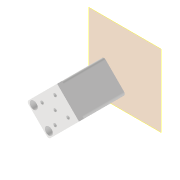
# Autodesk Inventor part: IM_ledmatrix_holder
Saved by Autodesk Inventor 2022 (Build 260153000, 153)
## iProperties
Created: 2023-06-20
Part Number: IM_ledmatrix_holder
Material: Generisch
Document SubType Name: Modeling
Designer: diederichbenedict
Density: 1 g/cm^3
Appearance: Vorgabe
Author: diederichbenedict
Autodesk Inventor part; units mm, degrees
ref_plane "YZ Plane" through (0, 0, 0) normal (1, 0, 0) x (0, 1, 0)
ref_plane "XZ Plane" through (0, 0, 0) normal (0, 1, 0) x (-1, 0, 0)
ref_plane "XY Plane" through (0, 0, 0) normal (0, 0, 1) x (1, 0, 0)
ref_plane "Arbeitsebene1" through (0, 0, 0) normal (0, 0, 1) x (1, 0, 0)
sketch "Skizze1" plane through (0, 0, 0) normal (0, 0, 1) x (1, 0, 0)
  circle A0 centre (-5.0971, -17.293) radius 1.4
  circle A1 centre (-17.4192, -5.2278) radius 1.4
  arc A2 (5.6957, 26.2674) -> (7.9686, 25.6694) centre (6.0612, 23.038) ccw
  arc A3 (5.6957, 26.2674) -> (-18.8161, -19.193) centre (0, 0) ccw
  arc A4 (-18.1702, -19.8055) -> (-18.8161, -19.193) centre (-16.2778, -17.1634) ccw
  arc A5 (-18.1702, -19.8055) -> (25.9554, 6.9811) centre (0, 0) ccw
  arc A6 (25.2463, 9.2218) -> (25.9554, 6.9811) centre (22.7119, 7.1872) ccw
  arc A7 (25.2463, 9.2218) -> (7.9686, 25.6694) centre (0, 0) ccw
  spline S0 degree 3 poles (-11.5553, -6.2972) (-11.3711, -6.4814) (-11.2247, -6.6998) (-11.0238, -7.1803) (-10.9713, -7.4379) (-10.9679, -7.9586) (-11.0171, -8.2168) (-11.2083, -8.6915) (-11.3454, -8.905) (-11.5184, -9.0874) knots 0 0 0 0 0.252225 0.252225 0.504373 0.504373 0.756494 0.756494 1 1 1 1
  line L0 (-11.5553, -6.2972) -> (-16.3497, -1.5028)
  arc A8 (-16.3497, 1.4985) -> (-16.3497, -1.5028) centre (-14.8491, -0.0022) ccw
  line L1 (-16.3497, 1.4985) -> (-1.5005, 16.3477)
  arc A9 (1.5007, 16.3477) -> (-1.5005, 16.3477) centre (0.0001, 14.8471) ccw
  line L2 (1.5007, 16.3477) -> (16.35, 1.4985)
  arc A10 (16.35, -1.5028) -> (16.35, 1.4985) centre (14.8494, -0.0022) ccw
  line L3 (16.35, -1.5028) -> (1.5007, -16.352)
  arc A11 (-1.5005, -16.352) -> (1.5007, -16.352) centre (0.0001, -14.8514) ccw
  line L4 (-1.5005, -16.352) -> (-4.7949, -13.0576)
  spline S1 degree 3 poles (-7.585, -13.0208) (-7.3961, -12.8415) (-7.1739, -12.7009) (-6.6882, -12.5128) (-6.4293, -12.4671) (-5.9087, -12.4775) (-5.6519, -12.5335) (-5.1824, -12.7372) (-4.9727, -12.8798) (-4.7949, -13.0576) knots 0 0 0 0 0.252231 0.252231 0.504388 0.504388 0.756517 0.756517 1 1 1 1
  arc A12 (-11.5184, -9.0874) -> (-7.585, -13.0208) centre (-9.4998, -11.0022) ccw
  line L5 (-17.4192, -5.2278) -> (-5.0971, -17.293)
  line L6 (-17.8503, -0.0022) -> (0.0001, -17.8526)
  line L7 (0.0001, -17.8526) -> (-3.889, -21.7417)
  line L8 (-6.7174, -21.7417) -> (-21.7394, -6.7197)
  line L9 (-21.7394, -3.8912) -> (-17.8503, -0.0022)
  arc A13 (-21.7394, -3.8912) -> (-21.7394, -6.7197) centre (-20.3252, -5.3055) ccw
  arc A14 (-6.7174, -21.7417) -> (-3.889, -21.7417) centre (-5.3032, -20.3275) ccw
  line L10 (-17.8503, -0.0022) -> (-18.5575, -0.7093)
  line L11 (-15.729, -0.7093) -> (-0.707, -15.7313)
  line L12 (-0.707, -18.5597) -> (0.0001, -17.8526)
  line L13 (0.0001, -17.8526) -> (-17.8503, -0.0022)
  arc A15 (-15.729, -0.7093) -> (-18.5575, -0.7093) centre (-17.1432, -2.1235) ccw
  arc A16 (-0.707, -18.5597) -> (-0.707, -15.7313) centre (-2.1212, -17.1455) ccw
  point P0 (0, 0)
  point P1 (-5.3032, -23.1559)
  point P2 (-11.5553, -6.2972)
  point P3 (-1.5005, -16.352)
  point P4 (-17.1432, 0.705)
  dimension "d0" = 7.5
  dimension "d1" = 2
  dimension "d23" = 1
  dimension "d24" = 2
  constraints: 18 end point, 8 point on circle, 8 tangent, 4 centre point, 4 parallel, 4 point on line, 3 perpendicular, 2 equal radius
  measures "d0" distance of L6.end point (-5.303, -23.156)
  measures "d1" radius of A13
  measures "d23" distance of L6.start point (-17.143, 0.705)
  measures "d24" radius of A15
extrude "Extrusion1" add sketch "Skizze1" along normal blind 50 contours L6 S1 A12 L5 S0 | S0 A12 S1 L4 L6 A16 L7 A14 L8 A13 L9 A15 L0 | L0 A8 A15 L11 A16 A11 L4 L6 | L6 A15 A8 | L5 A12 | A11 A16 L6
sketch "Skizze2" plane through (0, 0, 50) normal (0, 0, 1) x (1, 0, 0)
  line L0 (-21.2132, 0) -> (0, -21.2132) projected
  line L1 (-18.5575, -0.7093) -> (-21.7394, -3.8912) projected
  arc A0 (-21.7394, -3.8912) -> (-21.7394, -6.7197) centre (-20.3252, -5.3055) ccw projected
  line L2 (-21.7394, -6.7197) -> (-6.7174, -21.7417) projected
  arc A1 (-6.7174, -21.7417) -> (-3.889, -21.7417) centre (-5.3032, -20.3275) ccw projected
  line L3 (-3.889, -21.7417) -> (-0.707, -18.5597) projected
  circle A2 centre (-17.4192, -5.2278) radius 1.4 projected
  circle A3 centre (-5.0971, -17.293) radius 1.4 projected
  arc A4 (-0.707, -18.5597) -> (-0.707, -15.7313) centre (-2.1212, -17.1455) ccw projected
  line L4 (-0.707, -15.7313) -> (-15.729, -0.7093) projected
  arc A5 (-15.729, -0.7093) -> (-18.5575, -0.7093) centre (-17.1432, -2.1235) ccw projected
  point P0 (0, 0)
  point P1 (-1.6802, -19.533)
  point P2 (-3.7126, -17.5006)
  point P3 (-5.3048, -15.9084)
  point P4 (-16.0196, -5.1936)
  point P5 (-17.385, -3.8282)
  point P6 (-19.5307, -1.6825)
extrude "Extrusion2" add sketch "Skizze2" along normal blind 4 contours L0 A2 A3 L3 A1 L2 A0 L1
sketch "Skizze3" plane through (0, 0, 54) normal (0, 0, 1) x (1, 0, 0)
  line L0 (21.2132, 0) -> (0, 21.2132) projected
  line L1 (0, 21.2132) -> (-21.2132, 0) projected
  line L2 (-21.2132, 0) -> (0, -21.2132) projected
  line L3 (0, -21.2132) -> (21.2132, 0) projected
  circle A0 centre (0, 0) radius 1.3301 projected
  circle A1 centre (-10.6066, 0) radius 1.5 projected
  circle A2 centre (0, -10.6066) radius 1.5 projected
  circle A3 centre (10.6066, 0) radius 1.5 projected
  circle A4 centre (0, 10.6066) radius 1.5 projected
  line L4 (-3.889, -21.7417) -> (-1.6802, -19.533) projected
  line L5 (-1.6802, -19.533) -> (-3.7126, -17.5006) projected
  arc A5 (-5.3048, -15.9084) -> (-3.7126, -17.5006) centre (-5.0971, -17.293) ccw projected
  line L6 (-5.3048, -15.9084) -> (-16.0196, -5.1936) projected
  arc A6 (-17.385, -3.8282) -> (-16.0196, -5.1936) centre (-17.4192, -5.2278) ccw projected
  line L7 (-17.385, -3.8282) -> (-19.5307, -1.6825) projected
  line L8 (-19.5307, -1.6825) -> (-21.7394, -3.8912) projected
  arc A7 (-21.7394, -3.8912) -> (-21.7394, -6.7197) centre (-20.3252, -5.3055) ccw projected
  line L9 (-21.7394, -6.7197) -> (-6.7174, -21.7417) projected
  arc A8 (-6.7174, -21.7417) -> (-3.889, -21.7417) centre (-5.3032, -20.3275) ccw projected
  arc A9 (-16.0196, -5.1936) -> (-17.385, -3.8282) centre (-17.4192, -5.2278) ccw projected
  arc A10 (-3.7126, -17.5006) -> (-5.3048, -15.9084) centre (-5.0971, -17.293) ccw projected
  circle A11 centre (-10.6066, 0) radius 1.4
  circle A12 centre (0, 10.6066) radius 1.4
  circle A13 centre (10.6066, 0) radius 1.4
  circle A14 centre (0, -10.6066) radius 1.4
  line L10 (-19.5307, -1.6825) -> (1.6825, 19.5307)
  line L11 (-1.6802, -19.533) -> (19.533, 1.6802)
  point P0 (0, 0)
  dimension "d14" = 2.8
  dimension "d15" = 2.8
  dimension "d16" = 2.8
  dimension "d17" = 2.8
  constraints: 4 centre point, 4 coincident, 4 end point, 2 perpendicular, 2 point on line
  measures "d14" diameter of A11
  measures "d15" diameter of A12
  measures "d16" diameter of A13
  measures "d17" diameter of A14
extrude "Extrusion3" add sketch "Skizze3" along normal blind 4 contours L11 L2 A10 A9 L10 L0 | L4 A8 L9 A7 L8 L2 A6 A5 | A1 | A2 | A3 | A4
sketch "Skizze4" plane through (0.0001, -17.8526, 50) normal (0.7071068, -0.7071068, 0) x (-0.7071068, -0.7071068, 0)
  line L0 (5.5, 50) -> (1, 50) projected
  line L1 (2.3764, 0) -> (1, 0) projected
  line L2 (2.3764, 0) -> (2.3764, -4) projected
  line L3 (5.5, -8) -> (-27.6236, -8) projected
  line L4 (5.5, 50) -> (5.5, -8) projected
  line L5 (-2.5, 9.2593) -> (2.5, 9.2593)
  line L6 (2.5, 9.2593) -> (2.5, 12.2593)
  line L7 (2.5, 12.2593) -> (-2.5, 12.2593)
  line L8 (-2.5, 12.2593) -> (-2.5, 9.2593)
  line L9 (-2.5, 9.2593) -> (2.5, 12.2593) construction
  line L10 (2.5, 9.2593) -> (-2.5, 12.2593) construction
  line L11 (0, 9.2593) -> (2.5, 7.8159)
  line L12 (0, 9.2593) -> (2.8868, 9.2593) construction
  line L13 (2.5, 7.8159) -> (2.5, 13.7027)
  line L14 (2.5, 13.7027) -> (0, 12.2593)
  line L15 (2.3764, -4) -> (-27.6236, -4) projected
  line L16 (-27.6236, -4) -> (-27.6236, -8) projected
  line L17 (1, 50) -> (1, 0) projected
  point P0 (-12.6236, 50)
  point P1 (0, 10.7593)
  point P2 (2.5, 9.2593)
  dimension "d8" = 5
  dimension "d9" = 3
  dimension "d10" = 30
  dimension "d11" = 30
  constraints: 20 end point, 4 midpoint, 2 horizontal, 2 parallel, 1 equal length, 1 perpendicular
  measures "d8" distance of L7.end L6.end
  measures "d9" distance of L6.end L5.end
  measures "d10" angle of L11 L12
  measures "d11" angle of L7 L14
extrude "Extrusion4" cut sketch "Skizze4" against normal through all contours L7 L17 L5 L8 | L7 L6 L5 L17 | L17 L11 L5 | L5 L13 L11 L17
sketch "Skizze5" plane through (0, 0, 58) normal (0, 0, 1) x (1, 0, 0)
  circle A0 centre (-17.4192, -5.2278) radius 1.4 projected
  circle A1 centre (-5.0971, -17.293) radius 1.4 projected
  circle A2 centre (-17.4192, -5.2278) radius 3.25
  circle A3 centre (-5.0971, -17.293) radius 3.25
  point P0 (0, 0)
  dimension "d19" = 6.5
  dimension "d20" = 6.5
  constraints: 2 centre point, 2 coincident
  measures "d19" diameter of A2
  measures "d20" diameter of A3
extrude "Extrusion5" cut sketch "Skizze5" against normal blind 30 contours A0 | A1 | A2 | A3
sketch "Skizze6" plane through (-3.889, -21.7417, 58) normal (0.7071068, -0.7071068, 0) x (-0.7071068, -0.7071068, 0)
  line L0 (0.9585, 30) -> (-5.5415, 30) projected
  line L1 (-14.2171, 61.056) -> (6.1145, 61.056)
  line L2 (6.1145, 61.056) -> (6.1145, 38)
  line L3 (6.1145, 38) -> (-14.2171, 38)
  line L4 (-14.2171, 38) -> (-14.2171, 61.056)
  line L5 (0, 58) -> (-4.5, 58) projected
  point P0 (-18.1236, 58)
  dimension "d25" = 20
  constraints: 8 end point, 2 parallel, 1 horizontal, 1 perpendicular
  measures "d25" distance between parallel lines of L5 L3
extrude "Extrusion6" cut sketch "Skizze6" against normal blind 50
